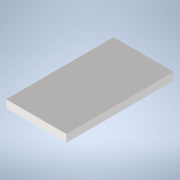
# Autodesk Inventor part: TTLUSB
Saved by Autodesk Inventor 2022 (Build 260153000, 153)
## iProperties
Created: 2021-11-04
Part Number: TTLUSB
Material: Generisch
Document SubType Name: Modeling
Designer: lukas
Density: 1 g/cm^3
Appearance: Vorgabe
Author: lukas
Autodesk Inventor part; units mm, degrees
ref_plane "YZ Plane" through (0, 0, 0) normal (1, 0, 0) x (0, 1, 0)
ref_plane "XZ Plane" through (0, 0, 0) normal (0, 1, 0) x (-1, 0, 0)
ref_plane "XY Plane" through (0, 0, 0) normal (0, 0, 1) x (1, 0, 0)
sketch "Skizze1" plane through (0, 0, 0) normal (0, 1, 0) x (-1, 0, 0)
  line L0 (0, 0) -> (-17.1, 0)
  line L1 (-17.1, 0) -> (-17.1, -30.6)
  line L2 (-17.1, -30.6) -> (0, -30.6)
  line L3 (0, -30.6) -> (0, 0)
  dimension "d0" = 17.1
  dimension "d1" = 30.6
  constraints: 8 end point, 2 parallel, 1 horizontal, 1 perpendicular
  measures "d0" distance of L2.end L1.end
  measures "d1" distance of L1.end L0.end
extrude "Extrusion1" add sketch "Skizze1" along normal blind 2.2
ref_plane "Arbeitsebene1" through (8.55, 0, -30.6) normal (-1, 0, 0) x (0, 0, 1)
